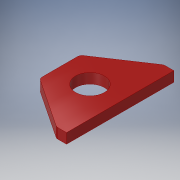
# Autodesk Inventor part: Limit Mount
Saved by Autodesk Inventor 2018.2 (Build 222227000, 227)
## iProperties
Created: 2018-01-30
Part Number: Limit Mount
Material: Steel
Document SubType Name: Modeling
Designer: torba
Density: 7.85 g/cm^3
Appearance: Red
Author: torba
Autodesk Inventor part; units mm, degrees
ref_plane "YZ Plane" through (0, 0, 0) normal (1, 0, 0) x (0, 1, 0)
ref_plane "XZ Plane" through (0, 0, 0) normal (0, 1, 0) x (-1, 0, 0)
ref_plane "XY Plane" through (0, 0, 0) normal (0, 0, 1) x (1, 0, 0)
sketch "Sketch1" plane through (0, 0, 0) normal (0, 1, 0) x (-1, 0, 0)
  line L0 (0, 0) -> (38.1, 0) construction
  line L1 (38.1, 0) -> (38.1, -25.4)
  line L2 (38.1, -25.4) -> (0, -25.4) construction
  line L3 (0, -25.4) -> (0, 0)
  line L4 (19.05, 0) -> (19.05, -25.4) construction
  line L5 (38.1, -12.7) -> (0, -12.7) construction
  circle A0 centre (19.05, -12.7) radius 9.0805
  line L6 (0, 0) -> (0, 25.4)
  line L7 (0, 25.4) -> (38.1, 0)
  line L8 (0, -25.4) -> (0, -50.8)
  line L9 (0, -50.8) -> (38.1, -25.4)
  dimension "d0" = 38.1
  dimension "d1" = 25.4
  dimension "d2" = 18.161
  dimension "d3" = 25.4
  dimension "d4" = 25.4
  constraints: 20 end point, 5 midpoint, 2 parallel, 1 centre point, 1 horizontal, 1 perpendicular, 1 point on line, 1 vertical
  measures "d0" distance of L1.end L2.end
  measures "d1" distance of L0.end L1.end
  measures "d2" diameter of A0
  measures "d3" distance of L0.start L6.end
  measures "d4" distance of L2.end L8.end
extrude "Extrusion1" add sketch "Sketch1" along normal blind 6.35
fillet "Fillet1" radius 3.175 2 edges at (-38.1, 3.175, 0) (-38.1, 3.175, -25.4)
sketch "Sketch2" plane through (0, 6.35, 0) normal (0, 1, 0) x (1, 0, 0)
  arc A0 (-36.6862, 26.3426) -> (-38.1, 23.7008) centre (-34.925, 23.7008) ccw projected
  line L0 (-38.1, 23.7008) -> (-38.1, 1.6992) projected
  arc A1 (-38.1, 1.6992) -> (-36.6862, -0.9426) centre (-34.925, 1.6992) ccw projected
  line L1 (-36.6862, -0.9426) -> (0, -25.4) projected
  line L2 (0, -25.4) -> (0, 50.8) projected
  line L3 (0, 50.8) -> (-36.6862, 26.3426) projected
  circle A2 centre (-19.05, 12.7) radius 9.0805 projected
  line L4 (0, -21.1667) -> (-6.35, -21.1667)
  line L5 (-36.6862, -0.9426) -> (0, -25.4) projected
  line L6 (0, -25.4) -> (0, 50.8) projected
  line L7 (0, 46.5667) -> (-6.35, 46.5667)
  line L8 (0, 50.8) -> (-36.6862, 26.3426) projected
  line L9 (0, 46.5667) -> (-12.9645, 46.5667)
  line L10 (-12.9645, 46.5667) -> (-12.9645, 61.1582)
  line L11 (-12.9645, 61.1582) -> (0, 61.1582)
  line L12 (0, 61.1582) -> (0, 46.5667)
  line L13 (0, -21.1667) -> (-12.9645, -21.1667)
  line L14 (-12.9645, -21.1667) -> (-12.9645, -45.9732)
  line L15 (-12.9645, -45.9732) -> (0, -45.9732)
  line L16 (0, -45.9732) -> (0, -21.1667)
  point P0 (0, 0)
  dimension "d8" = 6.35
  dimension "d9" = 6.35
  dimension "d10" = 25.1355
  dimension "d11" = 14.5915
  dimension "d12" = 107.1315
  constraints: 20 end point, 5 point on line, 4 horizontal, 4 parallel, 2 perpendicular
  measures "d8" distance of L4.start L4.end
  measures "d9" distance of L7.start L7.end
  measures "d10" distance between parallel lines of L0 L14
  measures "d11" distance between parallel lines of L11 L7
  measures "d12" distance between parallel lines of L11 L15
extrude "Extrusion2" cut sketch "Sketch2" against normal blind 6.35 contours L3 L2 L7 | L2 L1 L4
fillet "Fillet2" radius 3.175 2 edges at (-6.35, 3.175, 21.1667) (-6.35, 3.175, -46.5667)
body "Solid1"
